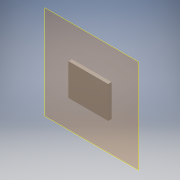
# Autodesk Inventor part: espaciador
Saved by Autodesk Inventor 2016 (Build 200138000, 138)
## iProperties
Created: 2017-02-23
Part Number: espaciador
Material: Generic
Document SubType Name: Modeling
Designer: jorge
Density: 1 g/cm^3
Appearance: Clear
Author: jorge
Autodesk Inventor part; units mm, degrees
ref_plane "YZ Plane" through (0, 0, 0) normal (1, 0, 0) x (0, 1, 0)
ref_plane "XZ Plane" through (0, 0, 0) normal (0, 1, 0) x (-1, 0, 0)
ref_plane "XY Plane" through (0, 0, 0) normal (0, 0, 1) x (1, 0, 0)
ref_plane "Work Plane1" through (0, 0, 0) normal (0, 0, 1) x (1, 0, 0)
sketch "Sketch1" plane through (0, 0, 0) normal (0, 0, 1) x (1, 0, 0)
  line L0 (17.5, -23.6854) -> (17.5, 23.6854) projected
  line L1 (-17.5, 23.6854) -> (-17.5, -23.6854) projected
  line L2 (17.5, 0) -> (17.5, 14)
  line L3 (17.5, 0) -> (17.5, -14)
  line L4 (17.5, 14) -> (-17.5, 14)
  line L5 (-17.5, 14) -> (-17.5, -14)
  line L6 (-17.5, -14) -> (17.5, -14)
  line L7 (17.5, -14) -> (17.5, 14)
  point P0 (0, 0)
  dimension "d0" = 14
  dimension "d1" = 14
  constraints: 12 end point, 3 point on line, 2 parallel, 1 horizontal, 1 midpoint, 1 perpendicular
  measures "d0" distance of L2.start L2.end
  measures "d1" distance of L2.start L3.end
extrude "Extrusion1" add sketch "Sketch1" along normal blind 3
sketch "Sketch2" plane through (0, 0, 0) normal (0, 0, -1) x (-1, 0, 0)
  circle A0 centre (5, -9) radius 1 projected
  circle A1 centre (-5, -9) radius 1 projected
  circle A2 centre (5, 9) radius 1 projected
  circle A3 centre (-5, 9) radius 1 projected
  point P0 (0, 0)
extrude "Extrusion2" cut sketch "Sketch2" against normal blind 3
body "Solid1"
